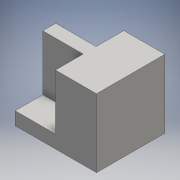
# Autodesk Inventor part: connectiontest1partB
Saved by Autodesk Inventor 2016 (Build 200138000, 138)
## iProperties
Created: 2015-11-20
Part Number: connectiontest1partB
Material: Generic
Document SubType Name: Modeling
Designer: hesaon
Density: 1 g/cm^3
Appearance: Default
Author: hesaon
Autodesk Inventor part; units mm, degrees
ref_plane "YZ Plane" through (0, 0, 0) normal (1, 0, 0) x (0, 1, 0)
ref_plane "XZ Plane" through (0, 0, 0) normal (0, 1, 0) x (-1, 0, 0)
ref_plane "XY Plane" through (0, 0, 0) normal (0, 0, 1) x (1, 0, 0)
sketch "Sketch1" plane through (0, 0, 0) normal (0, 0, 1) x (1, 0, 0)
  line L0 (0, 0) -> (23.8, 0)
  line L1 (23.8, 0) -> (23.8, 20)
  line L2 (23.8, 20) -> (0, 20)
  line L3 (0, 20) -> (0, 0)
  dimension "d0" = 23.8
  dimension "d1" = 20
  constraints: 8 end point, 2 parallel, 1 horizontal, 1 perpendicular
  measures "d0" distance of L2.end L1.end
  measures "d1" distance of L0.end L1.end
extrude "Extrusion1" add sketch "Sketch1" along normal blind 20
sketch "Sketch2" plane through (0, 0, 20) normal (0, 0, 1) x (1, 0, 0)
  line L0 (0, 0) -> (23.8, 0) projected
  line L1 (11.8, 0) -> (11.8, 8.1)
  line L2 (11.8, 8.1) -> (0, 8.1)
  line L3 (0, 8.1) -> (0, 11.9)
  line L4 (0, 20) -> (0, 0) projected
  line L5 (11.8, 11.9) -> (11.8, 20)
  line L6 (0, 11.9) -> (11.8, 11.9)
  line L7 (0, 0) -> (11.8, 0)
  dimension "d4" = 12
  dimension "d5" = 3.8
  dimension "d6" = 8.1
  dimension "d7" = 8.1
  dimension "d8" = 11.8
  constraints: 12 end point, 4 point on line, 3 perpendicular, 1 vertical
  measures "d4" distance of L0.end L1.start
  measures "d5" distance of L2.end L3.end
  measures "d6" distance of L0.start L2.end
  measures "d7" distance of L4.start L3.end
  measures "d8" distance of L4.start L5.end
extrude "Extrusion2" cut sketch "Sketch2" against normal blind 16.2 fills toward (5.9, 0.05) open curves L7 L1 L2 L3 L6 L5
sketch "Sketch3" plane through (0, 11.9, 20) normal (0, 1, 0) x (1, 0, 0)
  point P0 (0, 20)
body "Solid1"
